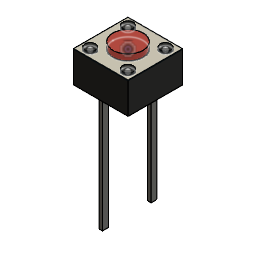
AlpsButton (Autodesk Fusion 360 design; units mm, degrees)
Autodesk Fusion 360 part; units mm, degrees
note: some values were not read from the file. Chosen so that the rebuilt part matches the saved one: which bodies a step acts on.
sketch "Sketch1" plane through (0, 0, 0) normal (0, 1, 0) x (1, 0, 0)
  line L0 (3.0988, -3.0861) -> (-3.0988, -3.0861)
  line L1 (-3.0988, -3.0861) -> (-3.0988, 3.0861)
  line L2 (-3.0988, 3.0861) -> (3.0988, 3.0861)
  line L3 (3.0988, 3.0861) -> (3.0988, -3.0861)
  line L4 (3.0988, -3.0861) -> (-3.0988, 3.0861) construction
  line L5 (-3.0988, -3.0861) -> (3.0988, 3.0861) construction
  dimension "d1" = 6.1976
  dimension "d2" = 6.1722
  constraint perpendicular L0 L1
  constraint parallel L0 L2
  constraint parallel L1 L3
  constraint horizontal L0
  constraint coincident L4 origin
  constraint coincident L5 origin
  measures "d1" distance of L1.end L2.end
  measures "d2" distance of L0.end L1.end
extrude "Extrude1" add sketch "Sketch1" along normal blind 3.5052 makes body 1
sketch "Sketch2" plane through (0, 3.5052, 0) normal (0, 1, 0) x (-1, 0, 0)
  line L0 (-3.0988, -3.0861) -> (3.0988, -3.0861)
  line L1 (3.0988, -3.0861) -> (3.0988, 3.0861)
  line L2 (3.0988, 3.0861) -> (-3.0988, 3.0861)
  line L3 (-3.0988, 3.0861) -> (-3.0988, -3.0861)
  circle A0 centre (0, 0) radius 1.7018
  circle A1 centre (2.0701, -2.0574) radius 0.5969
  circle A2 centre (-2.1971, -2.0574) radius 0.5969
  circle A3 centre (2.0701, 2.2098) radius 0.5969
  circle A4 centre (-2.1971, 2.2098) radius 0.5969
  dimension "d5" = 3.4036
  dimension "d8" = 1.1938
  dimension "d9" = 1.0287
  dimension "d10" = 1.0287
  dimension "d13" = -4.2672
  dimension "d14" = 4.2672
  constraint coincident A0.centre origin
  measures "d5" diameter of A0
  measures "d8" diameter of A1
  measures "d9" distance of L1 A1.centre
  measures "d10" distance of L0 A1.centre
extrude "Extrude2" add sketch "Sketch2" along normal blind 0.7366 contours A0 bodies 1
extrude "Extrude3" add sketch "Sketch2" along normal blind 0.2921 contours A1 | A2 | A3 | A4 bodies 1
sketch "Sketch3" plane through (0, 0, 0) normal (0, -1, 0) x (1, 0, 0)
  line L0 (-3.0988, -3.0861) -> (3.0988, -3.0861)
  line L1 (3.0988, -3.0861) -> (3.0988, 3.0861)
  line L2 (3.0988, 3.0861) -> (-3.0988, 3.0861)
  line L3 (-3.0988, 3.0861) -> (-3.0988, -3.0861)
  line L4 (-0.1905, 3.0861) -> (0.1905, 3.0861)
  line L5 (0.1905, 3.0861) -> (0.1905, 2.4257)
  line L6 (0.1905, 2.4257) -> (-0.1905, 2.4257)
  line L7 (-0.1905, 2.4257) -> (-0.1905, 3.0861)
  line L8 (-3.0988, 0) -> (3.0988, 0) construction
  line L9 (-0.1905, -2.4257) -> (-0.1905, -3.0861)
  line L10 (-0.1905, -3.0861) -> (0.1905, -3.0861)
  line L11 (0.1905, -3.0861) -> (0.1905, -2.4257)
  line L12 (0.1905, -2.4257) -> (-0.1905, -2.4257)
  dimension "d17" = 0.381
  dimension "d18" = 0.6604
  dimension "d19" = 0.1905
  constraint horizontal L4
  constraint vertical L5
  constraint horizontal L6
  constraint vertical L7
  constraint coincident L2 L4.start
  constraint midpoint L3 L8.start
  constraint midpoint L1 L8.end
  constraint symmetric L4.start L8 L9.end
  constraint symmetric L4.end L8 L10.end
  constraint symmetric L5.end L8 L11.end
  constraint symmetric L6.end L8 L9.start
  measures "d17" distance of L4.start L4.end
  measures "d18" distance of L4.start L6.end
  measures "d19" distance of origin L7
extrude "Extrude4" add sketch "Sketch3" along normal blind 12.7 contours L0 L9 L10 L11 L12 | L2 L4 L5 L6 L7 bodies 1
split "Split1" by plane through (0, 0, 0) normal (0, 1, 0) bodies 1 makes body 2 at (0.1905, -4.2333, 2.866) makes body 3 at (-2.1294, 0, 0.8086)
ref_plane "WorkPlane1" through (0, 3.5052, 0) normal (0, 1, 0) x (-1, 0, 0)
split "Split2" by plane through (0, 3.5052, 0) normal (0, 1, 0) bodies 3 makes body 4 at (-2.2536, 3.7973, 2.1801) makes body 5 at (0.6562, 4.2418, 0.5474) makes body 6 at (2.3037, 3.7973, -2.2696) makes body 7 at (-2.2536, 3.7973, -2.0871) makes body 8 at (2.3497, 3.7973, 2.5174)
extrude "Extrude5" add sketch "Sketch2" along normal blind 0.0508 bodies 3
split "Split3" by plane through (0, 3.5052, 0) normal (0, 1, 0) bodies 3 makes body 9 at (2.2801, 3.556, 0.0508)
equation "d1 = 0.244 \""
equation "d2 = 0.243 \""
equation "d3 = 0.138 \""
equation "d5 = 0.134 \""
equation "d6 = 0.029 \""
equation "d8 = 0.047 \""
equation "d9 = 0.0405 \""
equation "d10 = 0.0405 \""
equation "d13 = -0.168 \""
equation "d14 = 0.168 \""
equation "d15 = 0.0115 \""
equation "d17 = 0.015 \""
equation "d18 = 0.026 \""
equation "d19 = ( 0.015 / 2 ) * 1\""
equation "d20 = 0.5 \""
equation "d22 = 0.00 \""
equation "d23 = 0.002 \""
